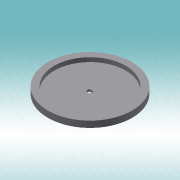
# Autodesk Inventor part: 計測輪20mm
Saved by Autodesk Inventor 2015 (Build 190159000, 159)
## iProperties
Created: 2016-04-10
Part Number: 計測輪20mm
Material: 一般
Document SubType Name: Modeling
Designer: buzztaka
Density: 1 g/cm^3
Appearance: 既定
Author: buzztaka
Autodesk Inventor part; units mm, degrees
ref_plane "YZ Plane" through (0, 0, 0) normal (1, 0, 0) x (0, 1, 0)
ref_plane "XZ Plane" through (0, 0, 0) normal (0, 1, 0) x (-1, 0, 0)
ref_plane "XY Plane" through (0, 0, 0) normal (0, 0, 1) x (1, 0, 0)
sketch "スケッチ1" plane through (0, 0, 0) normal (0, 0, 1) x (1, 0, 0)
  circle A0 centre (0, 0) radius 100
  dimension "d0" = 200
  constraints: 1 centre point, 1 coincident
  measures "d0" diameter of A0
extrude "押し出し1" add sketch "スケッチ1" along normal blind 15
sketch "スケッチ2" plane through (0, 0, 15) normal (0, 0, 1) x (1, 0, 0)
  circle A0 centre (0, 0) radius 85
  dimension "d3" = 170
  constraints: 1 centre point, 1 coincident
  measures "d3" diameter of A0
extrude "押し出し2" cut sketch "スケッチ2" against normal blind 10
sketch "スケッチ3" plane through (0, 0, 0) normal (0, 0, -1) x (-1, 0, 0)
  circle A0 centre (0, 0) radius 6
  dimension "d6" = 12
  constraints: 1 centre point, 1 coincident
  measures "d6" diameter of A0
extrude "押し出し3" cut sketch "スケッチ3" against normal through all
sketch "スケッチ4" plane through (0, 0, 5) normal (0, 0, 1) x (1, 0, 0)
  arc A0 (4.4721, 4) -> (-4.4721, 4) centre (0, 0) ccw
  line L0 (0, 4) -> (4.4721, 4)
  line L1 (0, 4) -> (-4.4721, 4)
  dimension "d9" = 12
  dimension "d10" = 4
  constraints: 4 end point, 2 point on circle, 1 centre point, 1 coincident, 1 horizontal, 1 point on line
  measures "d9" diameter of A0
  measures "d10" distance of point (0, 0) L0.start
extrude "押し出し4" add sketch "スケッチ4" against normal blind 5
